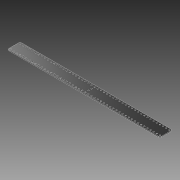
# Autodesk Inventor part: GreyT Claw Wide Plate V2
Saved by Autodesk Inventor 2022 (Build 260153000, 153)
## iProperties
Created: 2020-09-01
Part Number: GreyT Claw Wide Plate V2
Material: Aluminum 6061
Document SubType Name: Modeling
Density: 2.7 g/cm^3
Appearance: Glossy - Black
Autodesk Inventor part; units mm, degrees
ref_plane "YZ Plane" through (0, 0, 0) normal (1, 0, 0) x (0, 1, 0)
ref_plane "XZ Plane" through (0, 0, 0) normal (0, 1, 0) x (-1, 0, 0)
ref_plane "XY Plane" through (0, 0, 0) normal (0, 0, 1) x (1, 0, 0)
sketch "Sketch1" plane through (0, 0, 0) normal (0, 1, 0) x (-1, 0, 0)
  line L0 (-304.8, -25.4) -> (304.8, -25.4)
  line L1 (311.15, -19.05) -> (311.15, 19.05)
  line L2 (304.8, 25.4) -> (-304.8, 25.4)
  line L3 (-311.15, 19.05) -> (-311.15, -19.05)
  line L4 (-311.15, -25.4) -> (311.15, 25.4) construction
  line L5 (311.15, -25.4) -> (-311.15, 25.4) construction
  arc A0 (304.8, -25.4) -> (311.15, -19.05) centre (304.8, -19.05) ccw
  arc A1 (311.15, 19.05) -> (304.8, 25.4) centre (304.8, 19.05) ccw
  arc A2 (-311.15, -19.05) -> (-304.8, -25.4) centre (-304.8, -19.05) ccw
  arc A3 (-304.8, 25.4) -> (-311.15, 19.05) centre (-304.8, 19.05) ccw
  circle A4 centre (304.8, -19.05) radius 2.4892
  circle A5 centre (292.1, -19.05) radius 2.4892
  circle A6 centre (279.4, -19.05) radius 2.4892
  circle A7 centre (266.7, -19.05) radius 2.4892
  circle A8 centre (254, -19.05) radius 2.4892
  circle A9 centre (241.3, -19.05) radius 2.4892
  circle A10 centre (228.6, -19.05) radius 2.4892
  circle A11 centre (215.9, -19.05) radius 2.4892
  circle A12 centre (203.2, -19.05) radius 2.4892
  circle A13 centre (190.5, -19.05) radius 2.4892
  circle A14 centre (177.8, -19.05) radius 2.4892
  circle A15 centre (165.1, -19.05) radius 2.4892
  circle A16 centre (152.4, -19.05) radius 2.4892
  circle A17 centre (139.7, -19.05) radius 2.4892
  circle A18 centre (127, -19.05) radius 2.4892
  circle A19 centre (114.3, -19.05) radius 2.4892
  circle A20 centre (101.6, -19.05) radius 2.4892
  circle A21 centre (88.9, -19.05) radius 2.4892
  circle A22 centre (76.2, -19.05) radius 2.4892
  circle A23 centre (63.5, -19.05) radius 2.4892
  circle A24 centre (50.8, -19.05) radius 2.4892
  circle A25 centre (38.1, -19.05) radius 2.4892
  circle A26 centre (25.4, -19.05) radius 2.4892
  circle A27 centre (12.7, -19.05) radius 2.4892
  circle A28 centre (0, -19.05) radius 2.4892
  circle A29 centre (-12.7, -19.05) radius 2.4892
  circle A30 centre (-25.4, -19.05) radius 2.4892
  circle A31 centre (-38.1, -19.05) radius 2.4892
  circle A32 centre (-50.8, -19.05) radius 2.4892
  circle A33 centre (-63.5, -19.05) radius 2.4892
  circle A34 centre (-76.2, -19.05) radius 2.4892
  circle A35 centre (-88.9, -19.05) radius 2.4892
  circle A36 centre (-101.6, -19.05) radius 2.4892
  circle A37 centre (-114.3, -19.05) radius 2.4892
  circle A38 centre (-127, -19.05) radius 2.4892
  circle A39 centre (-139.7, -19.05) radius 2.4892
  circle A40 centre (-152.4, -19.05) radius 2.4892
  circle A41 centre (-165.1, -19.05) radius 2.4892
  circle A42 centre (-177.8, -19.05) radius 2.4892
  circle A43 centre (-190.5, -19.05) radius 2.4892
  circle A44 centre (-203.2, -19.05) radius 2.4892
  circle A45 centre (-215.9, -19.05) radius 2.4892
  circle A46 centre (-228.6, -19.05) radius 2.4892
  circle A47 centre (-241.3, -19.05) radius 2.4892
  circle A48 centre (-254, -19.05) radius 2.4892
  circle A49 centre (-266.7, -19.05) radius 2.4892
  circle A50 centre (-279.4, -19.05) radius 2.4892
  circle A51 centre (304.8, 19.05) radius 2.4892
  circle A52 centre (292.1, 19.05) radius 2.4892
  circle A53 centre (279.4, 19.05) radius 2.4892
  circle A54 centre (266.7, 19.05) radius 2.4892
  circle A55 centre (254, 19.05) radius 2.4892
  circle A56 centre (241.3, 19.05) radius 2.4892
  circle A57 centre (228.6, 19.05) radius 2.4892
  circle A58 centre (215.9, 19.05) radius 2.4892
  circle A59 centre (203.2, 19.05) radius 2.4892
  circle A60 centre (190.5, 19.05) radius 2.4892
  circle A61 centre (177.8, 19.05) radius 2.4892
  circle A62 centre (165.1, 19.05) radius 2.4892
  circle A63 centre (152.4, 19.05) radius 2.4892
  circle A64 centre (139.7, 19.05) radius 2.4892
  circle A65 centre (127, 19.05) radius 2.4892
  circle A66 centre (114.3, 19.05) radius 2.4892
  circle A67 centre (101.6, 19.05) radius 2.4892
  circle A68 centre (88.9, 19.05) radius 2.4892
  circle A69 centre (76.2, 19.05) radius 2.4892
  circle A70 centre (63.5, 19.05) radius 2.4892
  circle A71 centre (50.8, 19.05) radius 2.4892
  circle A72 centre (38.1, 19.05) radius 2.4892
  circle A73 centre (25.4, 19.05) radius 2.4892
  circle A74 centre (12.7, 19.05) radius 2.4892
  circle A75 centre (0, 19.05) radius 2.4892
  circle A76 centre (-12.7, 19.05) radius 2.4892
  circle A77 centre (-25.4, 19.05) radius 2.4892
  circle A78 centre (-38.1, 19.05) radius 2.4892
  circle A79 centre (-50.8, 19.05) radius 2.4892
  circle A80 centre (-63.5, 19.05) radius 2.4892
  circle A81 centre (-76.2, 19.05) radius 2.4892
  circle A82 centre (-88.9, 19.05) radius 2.4892
  circle A83 centre (-101.6, 19.05) radius 2.4892
  circle A84 centre (-114.3, 19.05) radius 2.4892
  circle A85 centre (-127, 19.05) radius 2.4892
  circle A86 centre (-139.7, 19.05) radius 2.4892
  circle A87 centre (-152.4, 19.05) radius 2.4892
  circle A88 centre (-165.1, 19.05) radius 2.4892
  circle A89 centre (-177.8, 19.05) radius 2.4892
  circle A90 centre (-190.5, 19.05) radius 2.4892
  circle A91 centre (-203.2, 19.05) radius 2.4892
  circle A92 centre (-215.9, 19.05) radius 2.4892
  circle A93 centre (-228.6, 19.05) radius 2.4892
  circle A94 centre (-241.3, 19.05) radius 2.4892
  circle A95 centre (-254, 19.05) radius 2.4892
  circle A96 centre (-266.7, 19.05) radius 2.4892
  circle A97 centre (-279.4, 19.05) radius 2.4892
  circle A98 centre (-292.1, -19.05) radius 2.4892
  circle A99 centre (-292.1, 19.05) radius 2.4892
  circle A100 centre (-304.8, -19.05) radius 2.4892
  circle A101 centre (-304.8, 19.05) radius 2.4892
  circle A102 centre (0, -6.35) radius 2.4892
  circle A103 centre (0, 6.35) radius 2.4892
  circle A104 centre (0, 19.05) radius 2.4892
  point P0 (0, 0)
  dimension "d0" = 622.3
  dimension "d1" = 50.8
  dimension "d2" = 6.35
  dimension "d5" = 12.7
  dimension "d8" = 38.1
  dimension "d13" = 12.7
  dimension "d18" = 4.9784
  constraints: 105 centre point, 12 end point, 8 point on circle, 8 point on line, 8 tangent, 3 equal radius, 2 horizontal, 2 midpoint, 2 parallel, 2 vertical, 1 coincident, 1 perpendicular, 200 other
  measures "d0" distance of L5.end L4.end
  measures "d1" distance of L4.end L5.start
  measures "d2" radius of A0
  measures "d5" distance of A4.centre A5.centre
  measures "d8" distance of A4.centre A51.centre
  measures "d13" distance of A28.centre A102.centre
  measures "d18" diameter of A4
extrude "Extrusion1" add sketch "Sketch1" along normal blind 3.175
body "Solid1"
